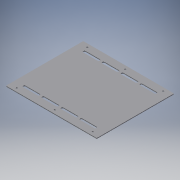
# Autodesk Inventor part: Deckel
Saved by Autodesk Inventor 2018 (Build 220112000, 112)
## iProperties
Created: 2017-11-12
Part Number: Deckel
Material: Generisch
Document SubType Name: Blech
Density: 1 g/cm^3
Sheet Metal Rule: Standard_mm
Appearance: Vorgabe
Flat Pattern Width: 22.4 cm
Flat Pattern Length: 26.3 cm
Flat Pattern Area: 589.12 cm^2
Sheet Metal Width: 224,000 mm
Sheet Metal Length: 263,000 mm
Sheet Metal Area: 58912,000 mm^2
Autodesk Inventor part; units mm, degrees
ref_plane "YZ Plane" through (0, 0, 0) normal (1, 0, 0) x (0, 1, 0)
ref_plane "XZ Plane" through (0, 0, 0) normal (0, 1, 0) x (-1, 0, 0)
ref_plane "XY Plane" through (0, 0, 0) normal (0, 0, 1) x (1, 0, 0)
sketch "Skizze1" plane through (0, 0, 0) normal (0, 0, 1) x (1, 0, 0)
  line L0 (-131.5, -112) -> (131.5, -112)
  line L1 (131.5, -112) -> (131.5, 112)
  line L2 (131.5, 112) -> (-131.5, 112)
  line L3 (-131.5, 112) -> (-131.5, -112)
  line L4 (-131.5, -112) -> (131.5, 112) construction
  line L5 (131.5, -112) -> (-131.5, 112) construction
  circle A0 centre (0, 102) radius 2.15
  line L6 (0, 156.8) -> (0, -156.8)
  circle A1 centre (-110, 102) radius 2.15
  circle A2 centre (110, 102) radius 2.15
  line L7 (-131.5, 0) -> (131.5, 0) construction
  circle A3 centre (0, -102) radius 2.15
  circle A4 centre (-110, -102) radius 2.15
  circle A5 centre (110, -102) radius 2.15
  point P0 (0, 0)
  dimension "d0" = 263
  dimension "d1" = 224
  dimension "d2" = 4.3
  dimension "d3" = 0
  dimension "d4" = 10
  dimension "d5" = 4.3
  dimension "d6" = 4.3
  dimension "d7" = 10
  dimension "d8" = 10
  dimension "d9" = 110
  dimension "d10" = 110
  measures "d0" distance of L2.end L1.end
  measures "d1" distance of L1.end L0.end
  measures "d2" diameter of A0
  measures "d3" distance from line of L6 A0.centre
  measures "d4" distance from line of L2 A0.centre
  measures "d5" diameter of A1
  measures "d6" diameter of A2
  measures "d7" distance from line of L2 A2.centre
  measures "d8" distance from line of L2 A1.centre
  measures "d9" distance of A0.centre A1.centre
  measures "d10" distance of A0.centre A2.centre
extrude "Grobblech1" add sketch "Skizze1" along normal blind 2 contours L3 L2 L6 A0 A3 L0 | L6 A3 A0 L2 L1 L0
fillet "Rundung1" radius 2 4 edges at (131.5, 112, 1) (131.5, -112, 1) (-131.5, -112, 1) (-131.5, 112, 1)
sketch "Skizze2" plane through (0, 0, 2) normal (0, 0, 1) x (1, 0, 0)
  arc A0 (-129.5, 112) -> (-131.5, 110) centre (-129.5, 110) ccw projected
  line L0 (-131.5, -110) -> (-131.5, 110) projected
  arc A1 (-131.5, -110) -> (-129.5, -112) centre (-129.5, -110) ccw projected
  line L1 (129.5, -112) -> (-129.5, -112) projected
  arc A2 (129.5, -112) -> (131.5, -110) centre (129.5, -110) ccw projected
  line L2 (131.5, 110) -> (131.5, -110) projected
  arc A3 (131.5, 110) -> (129.5, 112) centre (129.5, 110) ccw projected
  line L3 (-129.5, 112) -> (129.5, 112) projected
  circle A4 centre (110, -102) radius 2.15 projected
  circle A5 centre (0, -102) radius 2.15 projected
  circle A6 centre (-110, -102) radius 2.15 projected
  circle A7 centre (110, 102) radius 2.15 projected
  circle A8 centre (-110, 102) radius 2.15 projected
  circle A9 centre (0, 102) radius 2.15 projected
  line L4 (119.9374, -87) -> (-120.447, -87) construction
  line L5 (3.5, -87) -> (51.5, -87) construction
  line L6 (7, -90.5) -> (48, -90.5)
  line L7 (48, -83.5) -> (7, -83.5)
  arc A10 (7, -83.5) -> (7, -90.5) centre (7, -87) ccw
  arc A11 (48, -90.5) -> (48, -83.5) centre (48, -87) ccw
  line L8 (58.5, -87) -> (106.5, -87) construction
  line L9 (62, -90.5) -> (103, -90.5)
  line L10 (103, -83.5) -> (62, -83.5)
  arc A12 (62, -83.5) -> (62, -90.5) centre (62, -87) ccw
  arc A13 (103, -90.5) -> (103, -83.5) centre (103, -87) ccw
  line L11 (0, -102) -> (0, 102) construction
  line L12 (-327.71, -0.0001) -> (282.76, -0.0001) construction
  line L13 (-3.5, -87) -> (-51.5, -87) construction
  line L14 (-7, -90.5) -> (-48, -90.5)
  line L15 (-48, -83.5) -> (-7, -83.5)
  arc A14 (-7, -90.5) -> (-7, -83.5) centre (-7, -87) ccw
  arc A15 (-48, -83.5) -> (-48, -90.5) centre (-48, -87) ccw
  arc A16 (-62, -90.5) -> (-62, -83.5) centre (-62, -87) ccw
  line L16 (-62, -90.5) -> (-103, -90.5)
  line L17 (-103, -83.5) -> (-62, -83.5)
  line L18 (-58.5, -87) -> (-106.5, -87) construction
  arc A17 (-103, -83.5) -> (-103, -90.5) centre (-103, -87) ccw
  line L19 (3.5, 86.9998) -> (51.5, 86.9998) construction
  line L20 (7, 90.4998) -> (48, 90.4998)
  line L21 (48, 83.4998) -> (7, 83.4998)
  arc A18 (7, 90.4998) -> (7, 83.4998) centre (7, 86.9998) ccw
  arc A19 (48, 83.4998) -> (48, 90.4998) centre (48, 86.9998) ccw
  arc A20 (62, 90.4998) -> (62, 83.4998) centre (62, 86.9998) ccw
  line L22 (62, 90.4998) -> (103, 90.4998)
  line L23 (103, 83.4998) -> (62, 83.4998)
  line L24 (58.5, 86.9998) -> (106.5, 86.9998) construction
  arc A21 (103, 83.4998) -> (103, 90.4998) centre (103, 86.9998) ccw
  line L25 (-3.5, 86.9998) -> (-51.5, 86.9998) construction
  line L26 (-58.5, 86.9998) -> (-106.5, 86.9998) construction
  line L27 (-7, 90.4998) -> (-48, 90.4998)
  line L28 (-62, 90.4998) -> (-103, 90.4998)
  arc A22 (-7, 83.4998) -> (-7, 90.4998) centre (-7, 86.9998) ccw
  line L29 (-48, 83.4998) -> (-7, 83.4998)
  arc A23 (-48, 90.4998) -> (-48, 83.4998) centre (-48, 86.9998) ccw
  arc A24 (-62, 83.4998) -> (-62, 90.4998) centre (-62, 86.9998) ccw
  line L30 (-103, 83.4998) -> (-62, 83.4998)
  arc A25 (-103, 90.4998) -> (-103, 83.4998) centre (-103, 86.9998) ccw
  point P0 (0, 0)
  point P1 (65.6161, -112)
  point P2 (15.6161, -112)
  point P3 (-15.6161, -112)
  point P4 (-65.6161, -112)
  point P5 (5.6161, -112)
  point P6 (-5.6161, -112)
  point P7 (27.5, -87)
  point P8 (82.5, -87)
  point P9 (-119.9374, -87)
  point P10 (-27.5, -87)
  point P11 (-82.5, -87)
  point P12 (27.5, 86.9998)
  point P13 (82.5, 86.9998)
  point P14 (-27.5, 86.9998)
  point P15 (-82.5, 86.9998)
  dimension "d13" = 25
  dimension "d14" = 110
  dimension "d15" = 48
  dimension "d16" = 7
  dimension "d17" = 3.5
  dimension "d18" = 48
  dimension "d19" = 7
  dimension "d20" = 7
  dimension "d21" = 3.5
  constraints: 70 end point, 55 symmetric about line, 48 point on circle, 16 centre point, 16 point on line, 8 tangent, 2 midpoint, 2 parallel, 1 horizontal, 20 other
  measures "d13" distance between parallel lines of L1 L4
  measures "d14" distance of A5.centre A4.centre
  measures "d15" distance of L5.start L5.end
  measures "d16" diameter of A11
  measures "d17" horizontal distance of A5.centre L5.start
  measures "d18" distance of L8.start L8.end
  measures "d19" diameter of A13
  measures "d20" distance of L5.end L8.start
  measures "d21" horizontal distance of A4.centre L8.end
extrude "Extrusion1" cut sketch "Skizze2" against normal blind 10 contours A10 L7 A11 L6 | A12 L10 A13 L9 | L14 A15 L15 A14 | L16 A17 L17 A16 | L20 A19 L21 A18 | L22 A21 L23 A20 | A22 L29 A23 L27 | A24 L30 A25 L28
equation "\"d5\" = d2"
equation "\"d6\" = d2"
equation "\"d7\" = d4"
equation "\"d8\" = d4"
equation "\"d11\" = Stärke"
equation "\"Biegeradius\" = Stärke"
equation "\"BreiteBiegungsfreistellung\" = Stärke"
equation "\"TiefeBiegungsfreistellung\" = 0.5 * Stärke"
equation "\"GrößeEckenfreistellung\" = 4 * Stärke"
equation "\"MinimalRest\" = 2 * Stärke"
equation "\"Übergangsradius\" = Biegeradius"
equation "\"JacobiRadiusGröße\" = Biegeradius"
equation "\"Abstandsgröße\" = Stärke"
equation "\"Stärke\" = 2"
